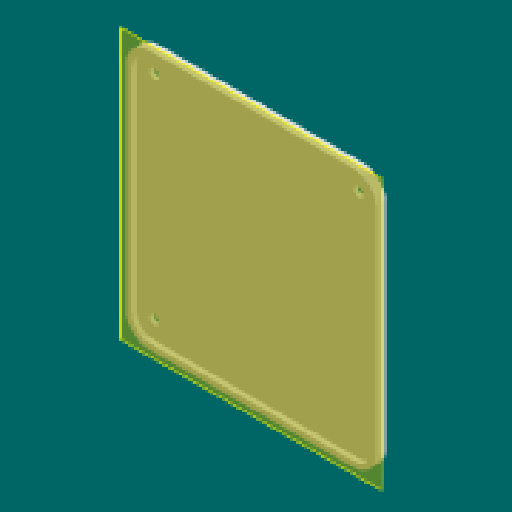
# Autodesk Inventor part: Part_atas
Saved by Autodesk Inventor 2025.2 (Build 292293000, 293)
## iProperties
Created: 2025-04-28
Part Number: Part_atas
Material: Generic
Document SubType Name: Modeling
Designer: ia088
Density: 1 g/cm^3
Appearance: Default
Author: ia088
Autodesk Inventor part; units mm, degrees
ref_plane "YZ Plane" through (0, 0, 0) normal (1, 0, 0) x (0, 1, 0)
ref_plane "XZ Plane" through (0, 0, 0) normal (0, 1, 0) x (-1, 0, 0)
ref_plane "XY Plane" through (0, 0, 0) normal (0, 0, 1) x (1, 0, 0)
ref_plane "Work Plane2" through (0, 0, 0) normal (0, 0, 1) x (1, 0, 0)
sketch "Sketch2" plane through (0, 0, 0) normal (0, 0, 1) x (1, 0, 0)
  line L0 (174.2186, -202.7504) -> (174.2186, -73.2206) projected
  arc A0 (184.2186, -63.2206) -> (174.2186, -73.2206) centre (184.2186, -73.2206) ccw projected
  circle A1 centre (184.2186, -73.2206) radius 3 projected
  line L1 (184.2186, -63.2206) -> (308.5414, -63.2206) projected
  circle A2 centre (308.5414, -73.2206) radius 3 projected
  arc A3 (318.5414, -73.2206) -> (308.5414, -63.2206) centre (308.5414, -73.2206) ccw projected
  line L2 (318.5414, -73.2206) -> (318.5414, -202.7504) projected
  arc A4 (308.5414, -212.7504) -> (318.5414, -202.7504) centre (308.5414, -202.7504) ccw projected
  line L3 (308.5414, -212.7504) -> (184.2186, -212.7504) projected
  arc A5 (174.2186, -202.7504) -> (184.2186, -212.7504) centre (184.2186, -202.7504) ccw projected
  circle A6 centre (184.2186, -202.7504) radius 3 projected
  circle A7 centre (308.5414, -202.7504) radius 3 projected
  line L4 (308.5414, -59.2206) -> (184.2186, -59.2206)
  arc A8 (184.2186, -59.2206) -> (170.2186, -73.2206) centre (184.2186, -73.2206) ccw
  line L5 (170.2186, -73.2206) -> (170.2186, -202.7504)
  arc A9 (170.2186, -202.7504) -> (184.2186, -216.7504) centre (184.2186, -202.7504) ccw
  line L6 (184.2186, -216.7504) -> (308.5414, -216.7504)
  arc A10 (308.5414, -216.7504) -> (322.5414, -202.7504) centre (308.5414, -202.7504) ccw
  line L7 (322.5414, -202.7504) -> (322.5414, -73.2206)
  arc A11 (322.5414, -73.2206) -> (308.5414, -59.2206) centre (308.5414, -73.2206) ccw
  arc A12 (184.2186, -63.7206) -> (174.7186, -73.2206) centre (184.2186, -73.2206) ccw
  point P0 (0, 0)
  dimension "d8" = 4
  constraints: 10 point on circle, 8 end point, 5 centre point, 7 other
  measures "d8" distance between parallel lines of L1 L4
ref_plane "Work Plane3" through (0, 0, 0) normal (0, 0, 1) x (1, 0, 0)
extrude "Extrusion3" add sketch "Sketch2" against normal blind 10 contours L0 A0 L1 A3 L2 A4 L3 A5 | A11 L7 A10 L6 A9 L5 A8 L4
sketch "Sketch4" plane through (0, 0, 0) normal (0, 0, 1) x (1, 0, 0)
  circle A0 centre (308.5414, -202.7504) radius 3 projected
  circle A1 centre (184.2186, -202.7504) radius 3 projected
  circle A2 centre (308.5414, -73.2206) radius 3 projected
  circle A3 centre (184.2186, -73.2206) radius 3 projected
  arc A4 (184.2186, -59.2206) -> (170.2186, -73.2206) centre (184.2186, -73.2206) ccw projected
  line L0 (170.2186, -73.2206) -> (170.2186, -202.7504) projected
  arc A5 (170.2186, -202.7504) -> (184.2186, -216.7504) centre (184.2186, -202.7504) ccw projected
  line L1 (184.2186, -216.7504) -> (308.5414, -216.7504) projected
  arc A6 (308.5414, -216.7504) -> (322.5414, -202.7504) centre (308.5414, -202.7504) ccw projected
  line L2 (322.5414, -202.7504) -> (322.5414, -73.2206) projected
  arc A7 (322.5414, -73.2206) -> (308.5414, -59.2206) centre (308.5414, -73.2206) ccw projected
  line L3 (308.5414, -59.2206) -> (184.2186, -59.2206) projected
  arc A8 (184.2186, -62.4206) -> (173.4186, -73.2206) centre (184.2186, -73.2206) ccw
  line L4 (173.4186, -73.2206) -> (173.4186, -202.7504)
  arc A9 (173.4186, -202.7504) -> (184.2186, -213.5504) centre (184.2186, -202.7504) ccw
  line L5 (184.2186, -213.5504) -> (308.5414, -213.5504)
  arc A10 (308.5414, -213.5504) -> (319.3414, -202.7504) centre (308.5414, -202.7504) ccw
  line L6 (319.3414, -202.7504) -> (319.3414, -73.2206)
  arc A11 (319.3414, -73.2206) -> (308.5414, -62.4206) centre (308.5414, -73.2206) ccw
  line L7 (308.5414, -62.4206) -> (184.2186, -62.4206)
  point P0 (0, 0)
  dimension "d10" = 3.2
  constraints: 8 end point, 8 point on circle, 4 centre point, 7 other
  measures "d10" distance between parallel lines of L3 L7
extrude "Extrusion4" cut sketch "Sketch4" against normal blind 7 contours L7 A11 L6 A10 L5 A9 L4 A8
sketch "Sketch5" plane through (0, 0, -10) normal (0, 0, -1) x (-1, 0, 0)
  circle A0 centre (-308.5414, -202.7504) radius 3 projected
  circle A1 centre (-184.2186, -202.7504) radius 3 projected
  circle A2 centre (-308.5414, -73.2206) radius 3 projected
  circle A3 centre (-184.2186, -73.2206) radius 3 projected
  circle A4 centre (-308.5414, -73.2206) radius 2.5
  circle A5 centre (-184.2186, -73.2206) radius 2.5
  circle A6 centre (-184.2186, -202.7504) radius 2.5
  circle A7 centre (-308.5414, -202.7504) radius 2.5
  point P0 (0, 0)
  dimension "d15" = 0.5
  dimension "d16" = 0.5
  dimension "d17" = 0.5
  dimension "d18" = 0.5
  constraints: 4 centre point
  measures "d15" radial gap between concentric circles of A2 A4
  measures "d16" radial gap between concentric circles of A3 A5
  measures "d17" radial gap between concentric circles of A1 A6
  measures "d18" radial gap between concentric circles of A0 A7
extrude "Extrusion5" add sketch "Sketch5" against normal up to surface (3 mm away)
sketch "Sketch6" plane through (0, 0, -10) normal (0, 0, -1) x (-1, 0, 0)
  circle A0 centre (-184.2186, -202.7504) radius 2.5 projected
  circle A1 centre (-308.5414, -73.2206) radius 2.5 projected
  circle A2 centre (-308.5414, -202.7504) radius 2.5 projected
  circle A3 centre (-184.2186, -73.2206) radius 2.5 projected
  point P0 (0, 0)
extrude "Extrusion6" add sketch "Sketch6" against normal blind 20.75
body "Solid1"
